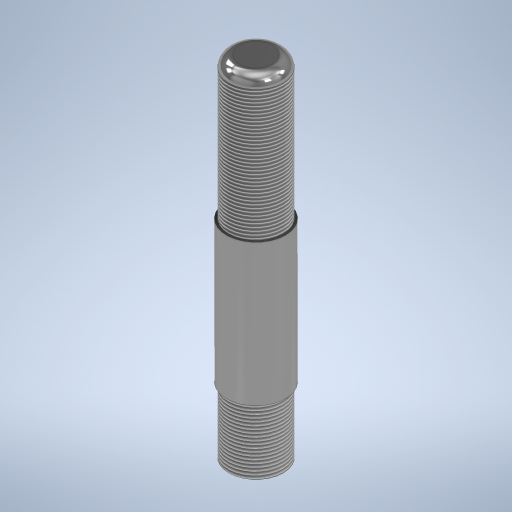
# Autodesk Inventor part: Stud
Saved by Autodesk Inventor 2024 (Build 280153000, 153)
## iProperties
Created: 2023-11-09
Part Number: Stud
Material: Steel, High Strength, Low Alloy
Document SubType Name: Modeling
Designer: Admin
Density: 7.85 g/cm^3
Appearance: Chrome - Polished Black
Author: Admin
Autodesk Inventor part; units mm, degrees
ref_plane "YZ Plane" through (0, 0, 0) normal (1, 0, 0) x (0, 1, 0)
ref_plane "XZ Plane" through (0, 0, 0) normal (0, 1, 0) x (-1, 0, 0)
ref_plane "XY Plane" through (0, 0, 0) normal (0, 0, 1) x (1, 0, 0)
sketch "Sketch1" plane through (0, 0, 0) normal (0, 1, 0) x (-1, 0, 0)
  circle A0 centre (0, 0) radius 13.5
  circle A1 centre (0, 0) radius 12.5
  dimension "d0" = 27
  dimension "d6" = 25
  constraints: 2 centre point, 2 coincident
  measures "d0" diameter of A0
  measures "d6" diameter of A1
extrude "Extrusion1" add sketch "Sketch1" along normal blind 160 contours A0 | A1
sketch "Sketch2" plane through (0, 160, 0) normal (0, 1, 0) x (1, 0, 0)
  circle A0 centre (0, 0) radius 13.5 projected
  circle A1 centre (0, 0) radius 12.5
  dimension "d3" = 25
  constraints: 1 centre point, 1 coincident
  measures "d3" diameter of A1
extrude "Extrusion2" cut sketch "Sketch2" against normal blind 65
extrude "Extrusion3" cut sketch "Sketch1" along normal blind 30
fillet "Fillet1" radius 5 1 edges at (-12.5, 160, 0)
thread "Thread1" size "M25x1.5" class "6g" standard "ANSI Metric M Profile" length 60
thread "Thread2" size "M25x1.5" class "6g" standard "ANSI Metric M Profile" length 30
body "Solid1"
